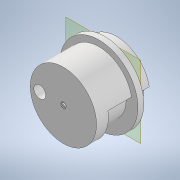
# Autodesk Inventor part: HandleGear2
Saved by Autodesk Inventor 2021 (Build 250183000, 183)
## iProperties
Created: 2021-03-29
Part Number: HandleGear2
Material: Generic
Document SubType Name: Modeling
Designer: ben
Density: 1 g/cm^3
Appearance: Default
Sheet Metal Rule: Default
Author: ben
Autodesk Inventor part; units mm, degrees
ref_plane "YZ Plane" through (0, 0, 0) normal (1, 0, 0) x (0, 1, 0)
ref_plane "XZ Plane" through (0, 0, 0) normal (0, 1, 0) x (-1, 0, 0)
ref_plane "XY Plane" through (0, 0, 0) normal (0, 0, 1) x (1, 0, 0)
sketch "Sketch1" plane through (0, 0, 0) normal (0, 0, 1) x (1, 0, 0)
  circle A0 centre (0.6539, 4.9671) radius 28 projected
  arc A1 (-24.346, 5.0297) -> (0.5914, -20.0328) centre (0.6539, 4.9671) ccw projected
  arc A2 (0.5914, -20.0328) -> (0.6164, -10.0328) centre (0.6039, -15.0328) ccw projected
  arc A3 (-14.346, 5.0047) -> (0.6164, -10.0328) centre (0.6539, 4.9671) ccw projected
  arc A4 (-14.346, 5.0047) -> (-24.346, 5.0297) centre (-19.346, 5.0172) ccw projected
  arc A5 (-3.34, -17.6834) -> (23.3045, 8.961) centre (0.6539, 4.9671) ccw
  line L0 (0.6539, 4.9671) -> (-3.34, -17.6834) construction
  line L1 (0.6539, 4.9671) -> (23.6539, 4.9671) construction
  line L2 (0.6539, 4.9671) -> (23.3045, 8.961) construction
  line L3 (-3.34, -17.6834) -> (-4.2082, -22.6075)
  line L4 (23.3045, 8.961) -> (28.2286, 9.8293)
  line L5 (3.5806, 5.6939) -> (3.546, 5.7006) projected
  line L6 (3.546, 5.7006) -> (-1.7356, 3.1802) projected
  line L7 (-1.7356, 3.1802) -> (-1.7521, 3.1491) projected
  arc A6 (-2.2009, 4.0894) -> (-1.7521, 3.1491) centre (0.6899, 4.8917) ccw projected
  line L8 (-2.2009, 4.0894) -> (-2.1663, 4.0827) projected
  line L9 (-2.1663, 4.0827) -> (3.1153, 6.6031) projected
  line L10 (3.1153, 6.6031) -> (3.1319, 6.6342) projected
  arc A7 (3.5806, 5.6939) -> (3.1319, 6.6342) centre (0.6899, 4.8917) ccw projected
  line L11 (-2.3009, 5.1265) -> (-1.5497, 4.6756) projected
  line L12 (-1.5497, 4.6756) -> (-2.2009, 4.0894) projected
  arc A8 (-2.3009, 5.1265) -> (-2.2009, 4.0894) centre (0.6899, 4.8917) ccw projected
  line L13 (-2.0402, 6.1352) -> (-1.4886, 5.4546) projected
  line L14 (-1.4886, 5.4546) -> (-2.3009, 5.1265) projected
  arc A9 (-2.0402, 6.1352) -> (-2.3009, 5.1265) centre (0.6899, 4.8917) ccw projected
  line L15 (-1.4503, 6.994) -> (-1.1647, 6.1657) projected
  line L16 (-1.1647, 6.1657) -> (-2.0402, 6.1352) projected
  arc A10 (-1.4503, 6.994) -> (-2.0402, 6.1352) centre (0.6899, 4.8917) ccw projected
  line L17 (-1.4503, 6.994) -> (-1.1647, 6.1657) projected
  line L18 (-1.1647, 6.1657) -> (-2.0402, 6.1352) projected
  arc A11 (-1.4503, 6.994) -> (-2.0402, 6.1352) centre (0.6899, 4.8917) ccw projected
  line L19 (-0.6171, 6.7232) -> (-1.4503, 6.994) projected
  arc A12 (-0.6022, 7.5992) -> (-1.4503, 6.994) centre (0.6899, 4.8917) ccw projected
  line L20 (-0.6022, 7.5992) -> (-0.6171, 6.7232) projected
  line L21 (0.0882, 7.0597) -> (-0.6022, 7.5992) projected
  arc A13 (0.4018, 7.8778) -> (-0.6022, 7.5992) centre (0.6899, 4.8917) ccw projected
  line L22 (0.4018, 7.8778) -> (0.0882, 7.0597) projected
  line L23 (0.866, 7.1347) -> (0.4018, 7.8778) projected
  arc A14 (1.4405, 7.7962) -> (0.4018, 7.8778) centre (0.6899, 4.8917) ccw projected
  line L24 (1.4405, 7.7962) -> (0.866, 7.1347) projected
  line L25 (1.6225, 6.9392) -> (1.4405, 7.7962) projected
  arc A15 (2.3886, 7.3644) -> (1.4405, 7.7962) centre (0.6899, 4.8917) ccw projected
  line L26 (2.3886, 7.3644) -> (1.6225, 6.9392) projected
  line L27 (3.1319, 6.6342) -> (2.2666, 6.4968) projected
  line L28 (2.2666, 6.4968) -> (2.3886, 7.3644) projected
  arc A16 (3.1319, 6.6342) -> (2.3886, 7.3644) centre (0.6899, 4.8917) ccw projected
  line L29 (3.6807, 4.6569) -> (2.9295, 5.1077) projected
  line L30 (2.9295, 5.1077) -> (3.5806, 5.6939) projected
  arc A17 (3.6807, 4.6569) -> (3.5806, 5.6939) centre (0.6899, 4.8917) ccw projected
  line L31 (2.8683, 4.3287) -> (3.6807, 4.6569) projected
  arc A18 (3.42, 3.6481) -> (3.6807, 4.6569) centre (0.6899, 4.8917) ccw projected
  line L32 (3.42, 3.6481) -> (2.8683, 4.3287) projected
  line L33 (2.5444, 3.6176) -> (3.42, 3.6481) projected
  arc A19 (2.83, 2.7893) -> (3.42, 3.6481) centre (0.6899, 4.8917) ccw projected
  line L34 (2.83, 2.7893) -> (2.5444, 3.6176) projected
  line L35 (1.9968, 3.0601) -> (2.83, 2.7893) projected
  arc A20 (1.9819, 2.1841) -> (2.83, 2.7893) centre (0.6899, 4.8917) ccw projected
  line L36 (1.9819, 2.1841) -> (1.9968, 3.0601) projected
  line L37 (1.2916, 2.7236) -> (1.9819, 2.1841) projected
  arc A21 (0.978, 1.9055) -> (1.9819, 2.1841) centre (0.6899, 4.8917) ccw projected
  line L38 (0.978, 1.9055) -> (1.2916, 2.7236) projected
  line L39 (0.5138, 2.6486) -> (0.978, 1.9055) projected
  arc A22 (-0.0607, 1.9871) -> (0.978, 1.9055) centre (0.6899, 4.8917) ccw projected
  line L40 (-0.0607, 1.9871) -> (0.5138, 2.6486) projected
  line L41 (-1.0089, 2.4189) -> (-0.2428, 2.8441) projected
  line L42 (-0.2428, 2.8441) -> (-0.0607, 1.9871) projected
  arc A23 (-1.0089, 2.4189) -> (-0.0607, 1.9871) centre (0.6899, 4.8917) ccw projected
  line L43 (-1.7521, 3.1491) -> (-0.8869, 3.2865) projected
  line L44 (-0.8869, 3.2865) -> (-1.0089, 2.4189) projected
  arc A24 (-1.7521, 3.1491) -> (-1.0089, 2.4189) centre (0.6899, 4.8917) ccw projected
  line L45 (0.6899, 4.8917) -> (-27.346, 4.8917)
  line L46 (-29.346, 4.8917) -> (-26.346, 6.6237)
  line L47 (-26.346, 6.6237) -> (-26.346, 3.1596)
  line L48 (-26.346, 3.1596) -> (-29.346, 4.8917)
  point P0 (0, 0)
  point P1 (-27.3183, 3.721)
  point P2 (-27.3248, 6.0586)
  point P3 (0.457, 4.0078)
  point P4 (0.2359, 5.229)
  point P5 (0.1644, 4.0869)
  point P6 (3.4147, 6.0323)
  point P7 (2.8549, 6.911)
  point P8 (2.8549, 6.911)
  point P9 (2.0283, 7.5453)
  point P10 (2.3889, 2.5701)
  point P11 (1.5148, 5.8393)
  point P12 (1.5561, 4.751)
  point P13 (2.3889, 2.5701)
  point P14 (-2.2181, 5.7864)
  point P15 (3.4147, 6.0323)
  point P16 (-2.3092, 4.9669)
  point P17 (2.0283, 7.5453)
  point P18 (1.48, 2.0033)
  point P19 (0.9312, 4.3735)
  point P20 (0.2466, 4.7001)
  point P21 (1.9636, 4.989)
  point P22 (1.6668, 4.939)
  point P23 (2.7913, 2.9016)
  point P24 (1.8206, 5.0572)
  point P25 (2.8045, 2.9146)
  point P26 (1.9816, 7.7503)
  point P27 (1.9816, 7.7503)
  point P28 (0.9776, 8.0288)
  point P29 (0.9776, 8.0288)
  point P30 (-0.0611, 7.9471)
  point P31 (-0.0611, 7.9471)
  point P32 (-1.0092, 7.5151)
  point P33 (-1.0092, 7.5151)
  point P34 (-1.7243, 3.2617)
  point P35 (3.6185, 5.2674)
  point P36 (3.6402, 5.0151)
  point P37 (0.0233, 4.8322)
  point P38 (-0.2672, 4.6867)
  point P39 (3.4147, 6.0323)
  point P40 (-2.3092, 4.9669)
  point P41 (-2.1379, 3.7591)
  point P42 (-1.555, 2.8426)
  point P43 (-2.3092, 4.9669)
  point P44 (0.4808, 4.8509)
  point P45 (2.9168, 3.4263)
  point P46 (-2.1989, 5.8449)
  point P47 (-0.2237, 5.0097)
  point P48 (0.5914, -20.0328)
  point P49 (0.6164, -10.0328)
  dimension "d8" = 23
  dimension "d9" = 100
  dimension "d10" = 110
  dimension "d11" = 4.924
  dimension "d12" = 4.924
  dimension "d18" = 3
  constraints: 18 end point, 5 point on circle, 2 horizontal, 1 centre point, 1 coincident, 1 equal length, 1 point on line, 7 other
  measures "d8" radius of A5
  measures "d9" angle of L0 L1
  measures "d10" angle of L0 L2
  measures "d11" horizontal distance of L2.end L4.end
  measures "d12" vertical distance of L0.end L3.end
  measures "d18" horizontal distance of L46.start L46.end
ref_plane "Work Plane1" through (-27.427, -23.1101, -9.6285) normal (0, 0, 1) x (0.9999965, 0.0026331, 0)
extrude "Extrusion3" add sketch "Sketch1" along normal blind -35 contours L4 A5 A2 A3 A4 A1 L45 L47 L46 A0 | A0 L48 L47 L45 A1 L3 | L46 L47 L45 A0 | A0 L48 L46 | A0 L45 L47 L48 | A1 L45 A3 A2 A5 L3 | A1 A4 A3 L45 | L30 L29 L31 L32 L33 L34 L35 L36 L37 L38 L39 L40 L42 L41 L44 L43 L7 L6 L5 | L5 L6 L7 A6 L8 L9 L10 A7 | A17 L29 L30 | L10 L9 L45 L11 L14 L13 L16 L15 L19 L20 L21 L22 L23 L24 L25 L26 L28 L27 | L27 L28 A16 | A18 L32 L31 | L26 L25 A15 | A19 L34 L33 | L43 L44 A24 | L9 L8 L12 L11 L45 | L24 L23 A14 | A20 L36 L35 | A8 L45 L11 L12 | L41 L42 A23 | L45 A8 L11 | L22 L21 A13 | A21 L38 L37 | L40 L39 A22 | A9 L13 L14 | L20 L19 A12 | A10 L15 L16
sketch "Sketch6" plane through (0, 0, 0) normal (0, 0, 1) x (-1, 0, 0)
  line L0 (-13, 18) -> (15, 18)
  line L1 (15, 18) -> (15, -27)
  line L2 (15, -27) -> (-13, -27)
  line L3 (-13, -27) -> (-13, 18)
  line L4 (26.346, -3.1596) -> (29.346, -4.8917) projected
  line L5 (29.346, -4.8917) -> (26.346, -6.6237) projected
  arc A0 (4.2082, 22.6075) -> (27.3183, -3.721) centre (-0.6539, -4.9671) ccw projected
  arc A1 (27.3248, -6.0586) -> (-28.2286, -9.8293) centre (-0.6539, -4.9671) ccw projected
  line L6 (-23.3045, -8.961) -> (-28.2286, -9.8293) projected
  arc A2 (-23.3045, -8.961) -> (3.34, 17.6834) centre (-0.6539, -4.9671) ccw projected
  line L7 (4.2082, 22.6075) -> (3.34, 17.6834) projected
  line L8 (2.0402, -6.1352) -> (1.4886, -5.4546) projected
  line L9 (1.4886, -5.4546) -> (2.3009, -5.1265) projected
  arc A3 (2.0402, -6.1352) -> (2.3009, -5.1265) centre (-0.6899, -4.8917) ccw projected
  line L10 (1.4503, -6.994) -> (1.1647, -6.1657) projected
  line L11 (1.1647, -6.1657) -> (2.0402, -6.1352) projected
  arc A4 (1.4503, -6.994) -> (2.0402, -6.1352) centre (-0.6899, -4.8917) ccw projected
  line L12 (0.6171, -6.7232) -> (1.4503, -6.994) projected
  arc A5 (0.6022, -7.5992) -> (1.4503, -6.994) centre (-0.6899, -4.8917) ccw projected
  line L13 (0.6022, -7.5992) -> (0.6171, -6.7232) projected
  line L14 (-0.0882, -7.0597) -> (0.6022, -7.5992) projected
  arc A6 (-0.4018, -7.8778) -> (0.6022, -7.5992) centre (-0.6899, -4.8917) ccw projected
  line L15 (-0.4018, -7.8778) -> (-0.0882, -7.0597) projected
  line L16 (-0.866, -7.1347) -> (-0.4018, -7.8778) projected
  arc A7 (-1.4405, -7.7962) -> (-0.4018, -7.8778) centre (-0.6899, -4.8917) ccw projected
  line L17 (-1.4405, -7.7962) -> (-0.866, -7.1347) projected
  line L18 (-1.6225, -6.9392) -> (-1.4405, -7.7962) projected
  arc A8 (-2.3886, -7.3644) -> (-1.4405, -7.7962) centre (-0.6899, -4.8917) ccw projected
  line L19 (-2.3886, -7.3644) -> (-1.6225, -6.9392) projected
  line L20 (-3.1319, -6.6342) -> (-2.2666, -6.4968) projected
  line L21 (-2.2666, -6.4968) -> (-2.3886, -7.3644) projected
  arc A9 (-3.1319, -6.6342) -> (-2.3886, -7.3644) centre (-0.6899, -4.8917) ccw projected
  line L22 (-2.5687, -6.3422) -> (1.6196, -4.3436) projected
  line L23 (-3.1153, -6.6031) -> (-2.5687, -6.3422) projected
  line L24 (1.6196, -4.3436) -> (2.1663, -4.0827) projected
  line L25 (1.7356, -3.1802) -> (1.1889, -3.4411) projected
  line L26 (1.1889, -3.4411) -> (-2.9993, -5.4397) projected
  line L27 (-2.9993, -5.4397) -> (-3.546, -5.7006) projected
  line L28 (-3.6807, -4.6569) -> (-2.9295, -5.1077) projected
  line L29 (-2.9295, -5.1077) -> (-3.5806, -5.6939) projected
  arc A10 (-3.6807, -4.6569) -> (-3.5806, -5.6939) centre (-0.6899, -4.8917) ccw projected
  line L30 (-2.8683, -4.3287) -> (-3.6807, -4.6569) projected
  arc A11 (-3.42, -3.6481) -> (-3.6807, -4.6569) centre (-0.6899, -4.8917) ccw projected
  line L31 (-3.42, -3.6481) -> (-2.8683, -4.3287) projected
  line L32 (-2.5444, -3.6176) -> (-3.42, -3.6481) projected
  arc A12 (-2.83, -2.7893) -> (-3.42, -3.6481) centre (-0.6899, -4.8917) ccw projected
  line L33 (-2.83, -2.7893) -> (-2.5444, -3.6176) projected
  line L34 (-1.9968, -3.0601) -> (-2.83, -2.7893) projected
  arc A13 (-1.9819, -2.1841) -> (-2.83, -2.7893) centre (-0.6899, -4.8917) ccw projected
  line L35 (-1.9819, -2.1841) -> (-1.9968, -3.0601) projected
  line L36 (-1.2916, -2.7236) -> (-1.9819, -2.1841) projected
  arc A14 (-0.978, -1.9055) -> (-1.9819, -2.1841) centre (-0.6899, -4.8917) ccw projected
  line L37 (-0.978, -1.9055) -> (-1.2916, -2.7236) projected
  line L38 (-0.5138, -2.6486) -> (-0.978, -1.9055) projected
  arc A15 (0.0607, -1.9871) -> (-0.978, -1.9055) centre (-0.6899, -4.8917) ccw projected
  line L39 (0.0607, -1.9871) -> (-0.5138, -2.6486) projected
  line L40 (1.0089, -2.4189) -> (0.2428, -2.8441) projected
  line L41 (0.2428, -2.8441) -> (0.0607, -1.9871) projected
  arc A16 (1.0089, -2.4189) -> (0.0607, -1.9871) centre (-0.6899, -4.8917) ccw projected
  line L42 (1.7521, -3.1491) -> (0.8869, -3.2865) projected
  line L43 (0.8869, -3.2865) -> (1.0089, -2.4189) projected
  arc A17 (1.7521, -3.1491) -> (1.0089, -2.4189) centre (-0.6899, -4.8917) ccw projected
  line L44 (2.3009, -5.1265) -> (1.5497, -4.6756) projected
  line L45 (1.5497, -4.6756) -> (2.2009, -4.0894) projected
  arc A18 (2.3009, -5.1265) -> (2.2009, -4.0894) centre (-0.6899, -4.8917) ccw projected
  line L46 (2.1663, -4.0827) -> (2.2009, -4.0894) projected
  line L47 (1.7521, -3.1491) -> (1.7356, -3.1802) projected
  line L48 (-3.1319, -6.6342) -> (-3.1153, -6.6031) projected
  line L49 (-3.546, -5.7006) -> (-3.5806, -5.6939) projected
  point P0 (0, 0)
  point P1 (15, -18.2483)
  point P2 (-13, -24.3727)
  point P3 (3.3958, 18)
  point P4 (27.3183, -3.721)
  point P5 (27.3248, -6.0586)
  point P6 (4.2082, 22.6075)
  point P7 (1.7988, -5.4825)
  point P8 (1.8856, -5.7173)
  point P9 (1.5854, -5.5741)
  point P10 (1.6812, -5.3768)
  point P11 (1.7057, -5.231)
  point P12 (1.7494, -5.3492)
  point P13 (1.0849, -5.3353)
  point P14 (1.267, -6.1621)
  point P15 (-3.0988, -6.512)
  point P16 (2.1543, -4.0884)
  point P17 (2.1652, -4.1215)
  point P18 (-2.3384, -3.7022)
  point P19 (1.6999, -5.3692)
  point P20 (1.8796, -4.8735)
  point P21 (2.1459, -4.1388)
  point P22 (-1.5148, -5.8393)
  point P23 (2.3092, -4.9669)
  point P24 (-2.1767, -6.1552)
  dimension "d27" = 28
  dimension "d28" = 45
  constraints: 8 end point, 2 parallel, 1 horizontal, 1 perpendicular
  measures "d27" distance of L1.end L2.end
  measures "d28" distance of L0.end L1.end
extrude "Extrusion6" add sketch "Sketch6" along normal blind 10 contours L3 A2 L6 A0 L7 L0 | L0 L7 A2 L1 L2 L3 | L7 A1 A0 L6 A2 L3 L2 L1 L0 | L0 L1 A2 L7 | A2 L2 L3 | L2 A2 | A2 L1 | A2 L1 L2 | L11 L10 L12 L13 L14 L15 L16 L17 L18 L19 L21 L20 L48 L23 L22 L24 L46 L45 L44 L9 L8 | L8 L9 A3 | A4 L10 L11 | L44 L45 A18 | A5 L13 L12 | A6 L15 L14 | A7 L17 L16 | A8 L19 L18 | A9 L20 L21 | L25 L26 L27 L49 L29 L28 L30 L31 L32 L33 L34 L35 L36 L37 L38 L39 L41 L40 L43 L42 L47 | L42 L43 A17 | L40 L41 A16 | L39 L38 A15 | A10 L28 L29 | L37 L36 A14 | A11 L31 L30 | L35 L34 A13 | A12 L33 L32
sketch "Sketch8" plane through (0, 0, 10) normal (0, 0, 1) x (-1, 0, 0)
  arc A0 (-0.5881, -29.9671) -> (24.346, -4.9013) centre (-0.6539, -4.9671) ccw projected
  arc A1 (24.346, -4.9013) -> (14.346, -4.9276) centre (19.346, -4.9145) ccw projected
  arc A2 (-0.6144, -19.9671) -> (14.346, -4.9276) centre (-0.6539, -4.9671) ccw projected
  circle A3 centre (19.346, -4.9145) radius 5
  point P0 (0, 0)
  point P1 (24.346, 4.9013)
  point P2 (-0.5881, 29.9671)
  point P3 (16.846, 4.9211)
  point P4 (15, 12.7905)
  point P5 (24.346, -4.9013)
  point P6 (16.8028, -0.6096)
  point P7 (15, 2.4422)
  point P8 (6.772, 18)
  point P9 (-0.6144, 19.9671)
  point P10 (21.6154, -0.4592)
  point P11 (24.346, -4.9145)
  point P12 (14.346, -4.9276)
  point P13 (24.346, -4.9013)
  constraints: 1 centre point, 1 coincident, 1 concentric
extrude "Extrusion7" cut sketch "Sketch8" against normal blind 20
ref_plane "Work Plane2" through (0, 0, -25) normal (0, 0, -1) x (1, 0, 0)
sketch "Sketch9" plane through (0, 0, -25) normal (0, 0, -1) x (1, 0, 0)
  arc A0 (27.4666, 3.1) -> (-19.297, -24.613) centre (0.6539, -4.9671) ccw projected
  arc A1 (-27.3183, -3.721) -> (-4.2082, 22.6075) centre (0.6539, -4.9671) ccw projected
  arc A2 (-19.297, -24.613) -> (27.4666, 3.1) centre (0.6539, -4.9671) ccw projected
  arc A3 (-31.9701, -9.9343) -> (33.278, -9.9343) centre (0.6539, -4.9671) ccw
  arc A4 (33.278, -9.9343) -> (-31.9701, -9.9343) centre (0.6539, -4.9671) ccw
  point P0 (0, 0)
  dimension "d34" = 5
  constraints: 4 point on circle, 2 centre point, 1 other
  measures "d34" radial gap between concentric circles of A2 A4
extrude "Extrusion8" add sketch "Sketch9" against normal blind 5 contours A1 A0 | A4 A3
sketch "Sketch10" plane through (0, 0, -35) normal (0, 0, -1) x (-1, 0, 0)
  circle A0 centre (-0.6539, 4.9671) radius 33 projected
  line L0 (6.8133, 16.1378) -> (5.2865, -7.085)
  line L1 (5.2865, -7.085) -> (-14.0617, 5.8487)
  line L2 (-14.0617, 5.8487) -> (6.8133, 16.1378)
  point P0 (0, 0)
  point P1 (-0.6539, 4.9671)
  dimension "d37" = 20.875
  constraints: 6 end point, 1 coincident, 7 other
  measures "d37" horizontal distance of L1.end L0.start
extrude "Extrusion9" cut sketch "Sketch10" against normal blind 15 contours L0 L1 L2
equation "\"BendRadius\" = Thickness"
equation "\"BendReliefWidth\" = Thickness"
equation "\"BendReliefDepth\" = 0.5 * Thickness"
equation "\"CornerReliefSize\" = 4 * Thickness"
equation "\"MinimumRemnant\" = 2 * Thickness"
equation "\"TransitionRadius\" = BendRadius"
equation "\"JacobiRadiusSize\" = Thickness"
equation "\"GapSize\" = Thickness"
equation "\"Thickness\" = 0.5"
body "Solid3"
